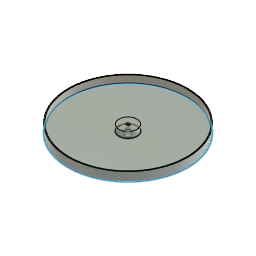
rotating_piece (Autodesk Fusion 360 design; units mm, degrees)
part number: 2025-11-03-16-37-40-676
Autodesk Fusion 360 part; units mm, degrees
note: some values were not read from the file. Set by a fixed rule: which sketch regions a step uses; the direction of a hole.
sketch "Boceto1" plane through (0, 0, 0) normal (0, 1, 0) x (1, 0, 0)
  circle A0 centre (100, -100) radius 100
extrude "Extruir1" add sketch "Boceto1" along normal blind 15
hole "Agujero1" at (100, 0, 100) direction (0, 1, 0) diameter 197 depth 197 tip angle 118
sketch "Boceto2" plane through (0, 0, 0) normal (0, 1, 0) x (1, 0, 0)
  circle A0 centre (100, -100) radius 100
  dimension "d6" = 200
  measures "d6" diameter of A0
extrude "Extruir2" cut sketch "Boceto1" along normal blind 0.003
extrude "Extruir3" add sketch "Boceto2" along normal blind 3
sketch "Boceto4" plane through (0, 3, 0) normal (0, 1, 0) x (-1, 0, 0)
  circle A0 centre (-100, 100) radius 98.5
  circle A1 centre (-100, 100) radius 15
  dimension "d11" = 30
  constraint concentric A0 A1
  measures "d11" diameter of A1
extrude "Extruir4" add sketch "Boceto4" along normal blind 10 contours A1
shell "Vaciado1" thickness 12 removed faces 1 at (101.1126, 13, 95.1254)
extrude "Extruir5" cut 1 faces at (98.8219, 12, 99.3198) along direction (0, -1, 0) blind 5
hole "Agujero2" at (100, 9.0986, 97) direction (0, 0, -1) diameter 5 depth 3 tip angle 118
sketch "Boceto5" plane through (0, 7, 0) normal (0, 1, 0) x (-1, 0, 0)
  circle A0 centre (-100, 100) radius 3
  line L0 (-97.7639, 98) -> (-102.2361, 98)
  constraint coincident A0 L0.end
  constraint coincident A0 L0.start
  constraint horizontal L0
extrude "Extruir6" add sketch "Boceto5" along normal blind 6 contours A0 L0 picked at (-100.6449, 97.9024)
sketch "Boceto6" plane through (0, 7, 0) normal (0, 1, 0) x (-1, 0, 0)
  line L0 (-102.2361, 98) -> (-97.7639, 98)
  arc A0 (-97.7639, 98) -> (-102.2361, 98) centre (-100, 100) ccw
  line L1 (-102.2361, 102) -> (-97.7639, 102)
  constraint coincident A0 L1.end
  constraint horizontal L1
  constraint coincident A0 L1.start
extrude "Extruir7" add sketch "Boceto6" along normal blind 6 contours A0 L1
